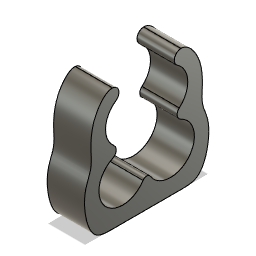
2 wire (ziptie) v2 (Autodesk Fusion 360 archive; units mm, degrees)
design "2 wire (ht)"
Autodesk Fusion 360 part; units mm, degrees
sketch "Sketch1" plane through (0, 0, 0) normal (1, 0, 0) x (0, 0, -1)
  arc A0 (-1.7252, -5.3917) -> (-2.3388, -5.3917) centre (-2.032, -5.5826) ccw
  arc A1 (-4.9259, -2.4778) -> (-4.8092, -1.5913) centre (-5.151, -1.9973) ccw
  arc A2 (-4.5933, 1.6761) -> (-4.8092, -1.5913) centre (-3.5004, -0.0369) ccw
  arc A3 (-4.5933, 1.6761) -> (-4.942, 2.7253) centre (-4.9853, 2.1284) ccw
  spline S0 degree 5 poles (-4.942, 2.7253) (-5.0108, 2.7298) (-5.1515, 2.719) (-5.3719, 2.6441) (-5.6787, 2.4311) (-6.0509, 2.0053) (-6.3722, 1.46) (-6.6087, 0.8412) (-6.7429, 0.1952) (-6.7866, -0.437) (-6.7727, -1.023) (-6.7432, -1.5409) (-6.7385, -1.983) (-6.7876, -2.3576) (-6.895, -2.6945) (-7.0391, -3.0399) (-7.1857, -3.4411) (-7.2967, -3.9334) (-7.3414, -4.5262) (-7.3057, -5.1888) (-7.189, -5.8659) (-6.9992, -6.4921) (-6.7492, -7.0069) (-6.4531, -7.3688) (-6.1219, -7.5724) (-5.7607, -7.6559) (-5.4492, -7.671) (-5.2026, -7.6764) (-5.0324, -7.6806) (-4.9459, -7.6828) knots 0 0 0 0 0 0 0.04 0.08 0.12 0.16 0.2 0.24 0.28 0.32 0.36 0.4 0.44 0.48 0.52 0.56 0.6 0.64 0.68 0.72 0.76 0.8 0.84 0.88 0.92 0.96 1 1 1 1 1 1
  line L0 (-4.3156, 2.6849) -> (-5.5683, 2.7657)
  line L1 (-6.1689, -7.651) -> (-3.7229, -7.7146)
  arc A4 (0.7452, -1.5913) -> (0.5215, 1.6811) centre (-0.5636, -0.0369) ccw
  arc A5 (0.7452, -1.5913) -> (0.8619, -2.4778) centre (1.087, -1.9973) ccw
  arc A6 (0.878, 2.7253) -> (0.5215, 1.6811) centre (0.9193, 2.1283) ccw
  arc A7 (-4.9259, -2.4778) -> (-2.3388, -5.3917) centre (-4.064, -4.318) ccw
  arc A8 (-1.7252, -5.3917) -> (0.8619, -2.4778) centre (0, -4.318) ccw
  spline S1 degree 5 poles (0.878, 2.7253) (0.9468, 2.7298) (1.0875, 2.719) (1.3079, 2.6441) (1.6147, 2.4311) (1.9869, 2.0053) (2.3082, 1.46) (2.5447, 0.8412) (2.6789, 0.1952) (2.7226, -0.437) (2.7087, -1.023) (2.6792, -1.5409) (2.6745, -1.983) (2.7236, -2.3576) (2.831, -2.6945) (2.9751, -3.0399) (3.1217, -3.4411) (3.2327, -3.9334) (3.2774, -4.5262) (3.2417, -5.1888) (3.125, -5.8659) (2.9352, -6.4921) (2.6852, -7.0069) (2.3891, -7.3688) (2.0579, -7.5724) (1.6967, -7.6559) (1.3852, -7.671) (1.1386, -7.6764) (0.9684, -7.6806) (0.8819, -7.6828) knots 0 0 0 0 0 0 0.04 0.08 0.12 0.16 0.2 0.24 0.28 0.32 0.36 0.4 0.44 0.48 0.52 0.56 0.6 0.64 0.68 0.72 0.76 0.8 0.84 0.88 0.92 0.96 1 1 1 1 1 1
  line L2 (0.2516, 2.6849) -> (1.5043, 2.7657)
  line L3 (2.1049, -7.651) -> (-0.3411, -7.7146)
  line L4 (-4.9459, -7.6828) -> (0.8819, -7.6828)
  point P0 (-6.604, 0.762)
  point P1 (-6.7719, -2.1775)
  point P2 (-7.2799, -3.9555)
  point P3 (-6.5179, -7.2575)
  point P4 (4.064, 0)
  point P5 (2.032, -5.5826)
  point P6 (4.064, 0)
  point P7 (2.032, -5.5826)
  point P8 (2.032, -5.2212)
  point P9 (1.7252, -5.3917)
  point P10 (2.54, 0.762)
  point P11 (2.7079, -2.1775)
  point P12 (3.2159, -3.9555)
  point P13 (2.4539, -7.2575)
  constraint midpoint A3.end L0
  constraint midpoint S0.end L1
  constraint horizontal L4
extrude "Extrude1" add sketch "Sketch1" along normal blind 3.175 in component "Component"
extrude "Extrude2" [suppressed]
extrude "Extrude1'" [suppressed]
fillet "Fillet1" [suppressed]
component "Component" placed x (1, 0, 0) y (0, 1, 0) z (0, 0, 1) at (0, 0, 0)
